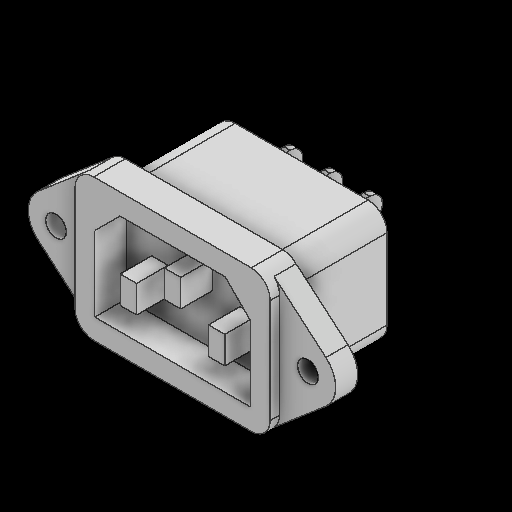
# Autodesk Inventor part: Qteatak
Saved by Autodesk Inventor 2025.2 (Build 292293000, 293)
## iProperties
Created: 2026-05-14
Part Number: Qteatak
Material: Generic
Document SubType Name: Modeling
Designer: valer
Density: 1 g/cm^3
Appearance: Default
Author: valer
Autodesk Inventor part; units mm, degrees
ref_plane "YZ Plane" through (0, 0, 0) normal (1, 0, 0) x (0, 1, 0)
ref_plane "XZ Plane" through (0, 0, 0) normal (0, 1, 0) x (-1, 0, 0)
ref_plane "XY Plane" through (0, 0, 0) normal (0, 0, 1) x (1, 0, 0)
sketch "Base" plane through (0, 0, 0) normal (0, 0, 1) x (1, 0, 0)
  line L0 (-12.5, -11.25) -> (12.5, -11.25)
  line L1 (15.5, -8.25) -> (15.5, 8.25)
  line L2 (12.5, 11.25) -> (-12.5, 11.25)
  line L3 (-15.5, 8.25) -> (-15.5, -8.25)
  line L4 (-15.5, -11.25) -> (15.5, 11.25) construction
  line L5 (15.5, -11.25) -> (-15.5, 11.25) construction
  line L6 (-34.16, 0) -> (34.16, 0) construction
  line L7 (0, -16.6198) -> (0, 16.6198) construction
  circle A0 centre (-20, 0) radius 1.65
  circle A1 centre (20, 0) radius 1.65
  circle A2 centre (-20, 0) radius 4.4
  circle A3 centre (20, 0) radius 4.4
  line L8 (-24.4, 0) -> (24.4, 0) construction
  arc A4 (-12.5, 11.25) -> (-15.5, 8.25) centre (-12.5, 8.25) ccw
  arc A5 (-15.5, -8.25) -> (-12.5, -11.25) centre (-12.5, -8.25) ccw
  arc A6 (15.5, 8.25) -> (12.5, 11.25) centre (12.5, 8.25) ccw
  arc A7 (12.5, -11.25) -> (15.5, -8.25) centre (12.5, -8.25) ccw
  line L9 (-22.8555, 3.3476) -> (-14.6213, 10.3713)
  line L10 (14.6213, 10.3713) -> (22.8555, 3.3476)
  line L11 (-22.8555, -3.3476) -> (-14.6213, -10.3713)
  line L12 (14.6213, -10.3713) -> (22.8555, -3.3476)
  point P0 (0, 0)
  dimension "d0" = 31
  dimension "d1" = 22.5
  dimension "d2" = 3.3
  dimension "d3" = 48.8
  dimension "d4" = 40
  dimension "d15" = 3
  dimension "d16" = 3
  constraints: 22 end point, 18 point on circle, 12 tangent, 11 point on line, 8 centre point, 3 equal radius, 2 coincident, 2 midpoint, 2 parallel, 1 horizontal, 1 perpendicular, 1 symmetric about line, 1 other
  measures "d0" distance of L4.start L5.start
  measures "d1" distance of L5.start L4.end
  measures "d2" diameter of A0
  measures "d3" distance of L8.end L8.start
  measures "d4" distance of A1.centre A0.centre
  measures "d15" radius of A4
  measures "d16" radius of A5
extrude "BaseFeature" add sketch "Base" along normal blind 3.5
sketch "ReceptacleInside" plane through (0, 0, 3.5) normal (0, 0, 1) x (1, 0, 0)
  line L0 (-12.35, 7.95) -> (12.35, 7.95)
  line L1 (12.35, 7.95) -> (12.35, -7.95)
  line L2 (12.35, -7.95) -> (-12.35, -7.95)
  line L3 (-12.35, -7.95) -> (-12.35, 7.95)
  line L4 (-12.35, 7.95) -> (12.35, -7.95) construction
  line L5 (12.35, 7.95) -> (-12.35, -7.95) construction
  line L6 (-12.35, 3.95) -> (-8.35, 7.95)
  line L7 (12.35, 3.95) -> (8.35, 7.95)
  line L8 (-34.16, 0) -> (34.16, 0) construction
  line L9 (0, -15.75) -> (0, 15.75) construction
  point P0 (0, 0)
  point P1 (8.35, 7.95)
  dimension "d10" = 15.9
  dimension "d11" = 4
  dimension "d12" = 4
  constraints: 16 end point, 4 midpoint, 2 parallel, 2 point on line, 1 horizontal, 1 perpendicular
  measures "d10" distance of L0.end L1.end
  measures "d11" distance of L0.start L6.end
  measures "d12" distance of L6.start L0.start
extrude "ReceptacleInsideFeature" cut sketch "ReceptacleInside" against normal through all contours L0 L7 L1 L2 L3 L6
sketch "Receptacle" plane through (0, 0, 3.5) normal (0, 0, 1) x (1, 0, 0)
  arc A0 (-12.5, 11.25) -> (-15.5, 8.25) centre (-12.5, 8.25) ccw projected
  line L0 (-15.5, 8.25) -> (-15.5, -8.25) projected
  arc A1 (-15.5, -8.25) -> (-12.5, -11.25) centre (-12.5, -8.25) ccw projected
  line L1 (-12.5, -11.25) -> (12.5, -11.25) projected
  arc A2 (12.5, -11.25) -> (15.5, -8.25) centre (12.5, -8.25) ccw projected
  line L2 (15.5, -8.25) -> (15.5, 8.25) projected
  arc A3 (15.5, 8.25) -> (12.5, 11.25) centre (12.5, 8.25) ccw projected
  line L3 (12.5, 11.25) -> (-12.5, 11.25) projected
  line L4 (-12.35, 3.95) -> (-8.35, 7.95) projected
  line L5 (-8.35, 7.95) -> (8.35, 7.95) projected
  line L6 (8.35, 7.95) -> (12.35, 3.95) projected
  line L7 (12.35, 3.95) -> (12.35, -7.95) projected
  line L8 (12.35, -7.95) -> (-12.35, -7.95) projected
  line L9 (-12.35, -7.95) -> (-12.35, 3.95) projected
  point P0 (0, 0)
extrude "Extrusion4" add sketch "Receptacle" along normal blind 1.5
sketch "Sketch5" plane through (0, 0, 0) normal (0, 0, -1) x (-1, 0, 0)
  line L0 (13.55, -9.35) -> (-13.55, -9.35)
  line L1 (-13.55, -9.35) -> (-13.55, 9.35)
  line L2 (-13.55, 9.35) -> (13.55, 9.35)
  line L3 (13.55, 9.35) -> (13.55, -9.35)
  line L4 (13.55, -9.35) -> (-13.55, 9.35) construction
  line L5 (-13.55, -9.35) -> (13.55, 9.35) construction
  point P0 (0, 0)
  dimension "d19" = 27.1
  dimension "d20" = 18.7
  constraints: 12 end point, 2 midpoint, 2 parallel, 1 horizontal, 1 perpendicular
  measures "d19" distance of L0.start L0.end
  measures "d20" distance of L0.end L1.end
extrude "Extrusion5" add sketch "Sketch5" along normal blind 15.5
fillet "Fillet1" radius 3 4 edges at (-13.55, -9.35, -7.75) (13.55, -9.35, -7.75) (-13.55, 9.35, -7.75) (13.55, 9.35, -7.75)
sketch "Sketch6" plane through (0, 0, 0) normal (0, 0, 1) x (1, 0, 0)
  line L0 (-34.16, 0) -> (34.16, 0) construction
  line L1 (-1.3, 0) -> (1.3, 0)
  line L2 (1.3, 0) -> (1.3, 4.33)
  line L3 (1.3, 4.33) -> (-1.3, 4.33)
  line L4 (-1.3, 4.33) -> (-1.3, 0)
  line L5 (0, -15.75) -> (0, 15.75) construction
  line L6 (-8.3, 0) -> (-5.7, 0)
  line L7 (-5.7, 0) -> (-5.7, -4.33)
  line L8 (-5.7, -4.33) -> (-8.3, -4.33)
  line L9 (-8.3, -4.33) -> (-8.3, 0)
  line L10 (8.3, 0) -> (5.7, 0)
  line L11 (5.7, 0) -> (5.7, -4.33)
  line L12 (5.7, -4.33) -> (8.3, -4.33)
  line L13 (8.3, -4.33) -> (8.3, 0)
  point P0 (0, 0)
  point P1 (7, -4.33)
  point P2 (-7, -4.33)
  dimension "d24" = 14
  dimension "d25" = 2.6
  dimension "d26" = 4.33
  constraints: 24 end point, 6 parallel, 4 symmetric about line, 3 midpoint, 2 horizontal, 2 perpendicular, 2 point on line
  measures "d24" distance of point (7, -4.33) point (-7, -4.33)
  measures "d25" distance from line of L7 L6.start
  measures "d26" distance of L3.end L1.start
extrude "Extrusion6" add sketch "Sketch6" along normal up to surface (5 mm away)
sketch "Sketch7" plane through (-10.55, -9.35, 0) normal (0, -1, 0) x (1, 0, 0)
  line L0 (0, -15.5) -> (21.1, -15.5) projected
  line L1 (3.72, -15.5) -> (4.72, -15.5)
  line L2 (4.72, -15.5) -> (4.72, -21.5)
  line L3 (4.72, -21.5) -> (3.72, -21.5)
  line L4 (3.72, -21.5) -> (3.72, -15.5)
  line L5 (10.05, -15.5) -> (11.05, -15.5)
  line L6 (11.05, -15.5) -> (11.05, -21.5)
  line L7 (11.05, -21.5) -> (10.05, -21.5)
  line L8 (10.05, -21.5) -> (10.05, -15.5)
  line L9 (16.38, -15.5) -> (17.38, -15.5)
  line L10 (17.38, -15.5) -> (17.38, -21.5)
  line L11 (17.38, -21.5) -> (16.38, -21.5)
  line L12 (16.38, -21.5) -> (16.38, -15.5)
  line L13 (10.55, -21.5) -> (10.55, 5) construction
  line L14 (11.85, 5) -> (9.25, 5) projected
  line L15 (10.55, -26.8) -> (10.55, 10.3) construction
  point P0 (10.55, 0)
  point P1 (4.72, -15.5)
  dimension "d29" = 6
  dimension "d30" = 5.33
  dimension "d31" = 5.33
  dimension "d32" = 1
  constraints: 26 end point, 6 parallel, 4 point on line, 3 equal length, 3 horizontal, 3 perpendicular, 2 midpoint, 1 collinear
  measures "d29" distance of L3.end L1.start
  measures "d30" distance between parallel lines of L8 L2
  measures "d31" distance between parallel lines of L12 L6
  measures "d32" distance between parallel lines of L2 L4
extrude "Extrusion7" add sketch "Sketch7" against normal up to surface (18.7 mm away)
sketch "Sketch8" plane through (6.83, -9.35, -15.5) normal (1, 0, 0) x (0, 0, -1)
  circle A0 centre (4, 5.35) radius 2
  line L0 (6, 0) -> (6, 18.7) projected
  line L1 (0, 0) -> (0, 18.7) projected
  line L2 (4, 3.35) -> (0, 3.35)
  line L3 (0, 3.35) -> (0, 7.35)
  line L4 (0, 7.35) -> (4, 7.35)
  line L5 (4, 7.35) -> (4, 3.35)
  line L6 (11.3, 9.35) -> (-25.8, 9.35) construction
  circle A1 centre (4, 13.35) radius 2
  line L7 (4, 15.35) -> (0, 15.35)
  line L8 (0, 11.35) -> (4, 11.35)
  line L9 (6, 18.7) -> (0, 18.7) projected
  line L10 (0, 0) -> (0, 18.7) projected
  line L11 (6, 0) -> (0, 0) projected
  line L12 (6, 0) -> (6, 18.7) projected
  point P0 (-15.5, 9.35)
  point P1 (6, 5.35)
  point P2 (0, 3.35)
  point P3 (6, 13.35)
  point P4 (0, 15.35)
  dimension "d35" = 4
  dimension "d36" = 4
  dimension "d37" = 4
  dimension "d38" = 2
  constraints: 12 end point, 5 symmetric about line, 4 point on circle, 2 centre point, 2 parallel, 1 horizontal, 1 perpendicular, 1 point on line, 1 tangent, 1 other
  measures "d35" diameter of A0
  measures "d36" distance between parallel lines of L4 L2
  measures "d37" distance of L2.start L2.end
  measures "d38" distance between parallel lines of L6 L4
extrude "Extrusion8" cut sketch "Sketch8" against normal through all contours L0 L11 L1 L2 A0 | A0 L4 L1 L8 A1 L0 | A1 L7 L1 L9 L0
equation "\"d27\" = d25"
equation "\"d33\" = d30"
body "Solid1"
